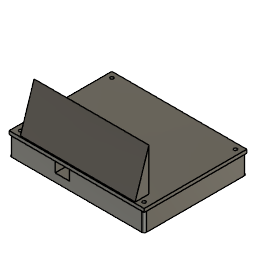
inky_case (Autodesk Fusion 360 design; units mm, degrees)
Autodesk Fusion 360 part; units mm, degrees
sketch "Sketch1" plane through (0, 0, 0) normal (0, 0, 1) x (1, 0, 0)
  line L0 (-58.8, -44.75) -> (58.8, -44.75)
  line L1 (58.8, -44.75) -> (58.8, 44.75)
  line L2 (58.8, 44.75) -> (-58.8, 44.75)
  line L3 (-58.8, 44.75) -> (-58.8, -44.75)
extrude "Extrude1" add sketch "Sketch1" along normal blind 16 makes body 1
ref_plane "WorkPlane1" through (0, 0, 2) normal (0, 0, 1) x (1, 0, 0)
sketch "Sketch2" plane through (0, 0, 2) normal (0, 0, 1) x (1, 0, 0)
  line L0 (-48.8, -34.75) -> (48.8, -34.75)
  line L1 (48.8, -34.75) -> (48.8, 34.75)
  line L2 (48.8, 34.75) -> (-48.8, 34.75)
  line L3 (-48.8, 34.75) -> (-48.8, -34.75)
extrude "Extrude2" add sketch "Sketch2" along normal blind 15 separate body makes body 2
combine "Combine1" operation cut target body 1 tool bodies 2
ref_plane "WorkPlane2" through (0, 0, -1) normal (0, 0, 1) x (1, 0, 0)
sketch "Sketch3" plane through (0, 0, -1) normal (0, 0, 1) x (1, 0, 0)
  line L0 (-43, -24.35) -> (43, -24.35)
  line L1 (43, -24.35) -> (43, 29.65)
  line L2 (43, 29.65) -> (-43, 29.65)
  line L3 (-43, 29.65) -> (-43, -24.35)
extrude "Extrude3" add sketch "Sketch3" along normal blind 4 separate body makes body 3
combine "Combine2" operation cut target body 1 tool bodies 3
ref_plane "WorkPlane3" through (0, -45.25, 0) normal (0, 1, 0) x (0, 0, 1)
sketch "Sketch4" plane through (0, -45.25, 0) normal (0, 1, 0) x (1, 0, 0)
  line L0 (-18.7, -7.2) -> (-6.3, -7.2)
  line L1 (-6.3, -7.2) -> (-6.3, -17.8)
  line L2 (-6.3, -17.8) -> (-18.7, -17.8)
  line L3 (-18.7, -17.8) -> (-18.7, -7.2)
extrude "Extrude4" add sketch "Sketch4" along normal blind 11 separate body makes body 4
combine "Combine3" operation cut target body 1 tool bodies 4
ref_plane "WorkPlane4" through (0, 0, 11) normal (0, 0, 1) x (1, 0, 0)
sketch "Sketch5" plane through (0, 0, 11) normal (0, 0, 1) x (1, 0, 0)
  circle A0 centre (-53.8, -39.75) radius 1
extrude "Extrude5" add sketch "Sketch5" along normal blind 5 separate body makes body 5
combine "Combine4" operation cut target body 1 tool bodies 5
ref_plane "WorkPlane5" through (0, 0, 11) normal (0, 0, 1) x (1, 0, 0)
sketch "Sketch6" plane through (0, 0, 11) normal (0, 0, 1) x (1, 0, 0)
  circle A0 centre (-53.8, 39.75) radius 1
extrude "Extrude6" add sketch "Sketch6" along normal blind 5 separate body makes body 6
combine "Combine5" operation cut target body 1 tool bodies 6
ref_plane "WorkPlane6" through (0, 0, 11) normal (0, 0, 1) x (1, 0, 0)
sketch "Sketch7" plane through (0, 0, 11) normal (0, 0, 1) x (1, 0, 0)
  circle A0 centre (53.8, -39.75) radius 1
extrude "Extrude7" add sketch "Sketch7" along normal blind 5 separate body makes body 7
combine "Combine6" operation cut target body 1 tool bodies 7
ref_plane "WorkPlane7" through (0, 0, 11) normal (0, 0, 1) x (1, 0, 0)
sketch "Sketch8" plane through (0, 0, 11) normal (0, 0, 1) x (1, 0, 0)
  circle A0 centre (53.8, 39.75) radius 1
extrude "Extrude8" add sketch "Sketch8" along normal blind 5 separate body makes body 8
combine "Combine7" operation cut target body 1 tool bodies 8
fillet "Fillet1" radius 2 4 edges at (-58.8, -44.75, 8) (58.8, -44.75, 8) (-58.8, 44.75, 8) (58.8, 44.75, 8) on bodies 1
ref_plane "WorkPlane8" through (0, 0, -0.5) normal (0, 0, 1) x (1, 0, 0)
sketch "Sketch9" plane through (0, 0, -0.5) normal (0, 0, 1) x (1, 0, 0)
  line L0 (-34.2331, 31.33) -> (-32.5755, 32.1283)
  line L1 (-32.5755, 32.1283) -> (-31.2436, 30.8591)
  line L2 (-31.2436, 30.8591) -> (-31.4906, 32.6823)
  line L3 (-31.4906, 32.6823) -> (-29.8719, 33.5569)
  line L4 (-29.8719, 33.5569) -> (-31.6822, 33.8853)
  line L5 (-31.6822, 33.8853) -> (-32.0138, 35.695)
  line L6 (-32.0138, 35.695) -> (-32.8856, 34.0748)
  line L7 (-32.8856, 34.0748) -> (-34.7092, 34.3187)
  line L8 (-34.7092, 34.3187) -> (-33.4377, 32.9889)
  line L9 (-33.4377, 32.9889) -> (-34.2331, 31.33)
extrude "Extrude9" add sketch "Sketch9" along normal blind 1.1 separate body makes body 9
combine "Combine8" operation cut target body 1 tool bodies 9
ref_plane "WorkPlane9" through (0, 0, -0.5) normal (0, 0, 1) x (1, 0, 0)
sketch "Sketch10" plane through (0, 0, -0.5) normal (0, 0, 1) x (1, 0, 0)
  circle A0 centre (-17.7225, 35.7912) radius 2.0607
  circle A1 centre (-16.9103, 35.6895) radius 2.0607
extrude "Extrude10" add sketch "Sketch10" along normal blind 1.1 separate body contours A0 A1 picked at (-19.4686, 36.1615) makes body 10
combine "Combine9" operation cut target body 1 tool bodies 10
ref_plane "WorkPlane10" through (0, 0, -0.5) normal (0, 0, 1) x (1, 0, 0)
sketch "Sketch11" plane through (0, 0, -0.5) normal (0, 0, 1) x (1, 0, 0)
  line L0 (-6.1051, 39.8174) -> (-6.8302, 37.9206)
  line L1 (-6.8302, 37.9206) -> (-8.853, 38.0986)
  line L2 (-8.853, 38.0986) -> (-7.2731, 36.8229)
  line L3 (-7.2731, 36.8229) -> (-8.0675, 34.954)
  line L4 (-8.0675, 34.954) -> (-6.366, 36.0624)
  line L5 (-6.366, 36.0624) -> (-4.834, 34.7294)
  line L6 (-4.834, 34.7294) -> (-5.3624, 36.6902)
  line L7 (-5.3624, 36.6902) -> (-3.6213, 37.7352)
  line L8 (-3.6213, 37.7352) -> (-5.6493, 37.8386)
  line L9 (-5.6493, 37.8386) -> (-6.1051, 39.8174)
extrude "Extrude11" add sketch "Sketch11" along normal blind 1.1 separate body makes body 11
combine "Combine10" operation cut target body 1 tool bodies 11
ref_plane "WorkPlane11" through (0, 0, -0.5) normal (0, 0, 1) x (1, 0, 0)
sketch "Sketch12" plane through (0, 0, -0.5) normal (0, 0, 1) x (1, 0, 0)
  line L0 (8.0648, 38.7951) -> (8.2392, 36.9319)
  line L1 (8.2392, 36.9319) -> (6.6062, 36.0181)
  line L2 (6.6062, 36.0181) -> (8.432, 35.6083)
  line L3 (8.432, 35.6083) -> (8.7965, 33.7728)
  line L4 (8.7965, 33.7728) -> (9.7505, 35.3826)
  line L5 (9.7505, 35.3826) -> (11.6087, 35.1621)
  line L6 (11.6087, 35.1621) -> (10.3725, 36.5669)
  line L7 (10.3725, 36.5669) -> (11.1565, 38.266)
  line L8 (11.1565, 38.266) -> (9.4385, 37.5244)
  line L9 (9.4385, 37.5244) -> (8.0648, 38.7951)
extrude "Extrude12" add sketch "Sketch12" along normal blind 1.1 separate body makes body 12
combine "Combine11" operation cut target body 1 tool bodies 12
ref_plane "WorkPlane12" through (0, 0, -0.5) normal (0, 0, 1) x (1, 0, 0)
sketch "Sketch13" plane through (0, 0, -0.5) normal (0, 0, 1) x (1, 0, 0)
  circle A0 centre (25.2651, 33.3164) radius 2.102
  circle A1 centre (24.8487, 32.1532) radius 2.102
extrude "Extrude13" add sketch "Sketch13" along normal blind 1.1 separate body contours A0 A1 picked at (26.0223, 34.8247) makes body 13
combine "Combine12" operation cut target body 1 tool bodies 13
ref_plane "WorkPlane13" through (0, 0, -0.5) normal (0, 0, 1) x (1, 0, 0)
sketch "Sketch14" plane through (0, 0, -0.5) normal (0, 0, 1) x (1, 0, 0)
  line L0 (43.3477, 37.6323) -> (44.4797, 38.9174)
  line L1 (44.4797, 38.9174) -> (46.1221, 38.4324)
  line L2 (46.1221, 38.4324) -> (45.2497, 39.9061)
  line L3 (45.2497, 39.9061) -> (46.2186, 41.3182)
  line L4 (46.2186, 41.3182) -> (44.5474, 40.9439)
  line L5 (44.5474, 40.9439) -> (43.5038, 42.3017)
  line L6 (43.5038, 42.3017) -> (43.3433, 40.5967)
  line L7 (43.3433, 40.5967) -> (41.7295, 40.0237)
  line L8 (41.7295, 40.0237) -> (43.3015, 39.3443)
  line L9 (43.3015, 39.3443) -> (43.3477, 37.6323)
extrude "Extrude14" add sketch "Sketch14" along normal blind 1.1 separate body makes body 14
combine "Combine13" operation cut target body 1 tool bodies 14
ref_plane "WorkPlane14" through (0, 0, -0.5) normal (0, 0, 1) x (1, 0, 0)
sketch "Sketch15" plane through (0, 0, -0.5) normal (0, 0, 1) x (1, 0, 0)
  line L0 (43.5729, 24.2177) -> (45.2148, 23.1167)
  line L1 (45.2148, 23.1167) -> (44.5685, 21.2483)
  line L2 (44.5685, 21.2483) -> (46.1231, 22.4697)
  line L3 (46.1231, 22.4697) -> (47.7003, 21.2777)
  line L4 (47.7003, 21.2777) -> (47.0191, 23.1336)
  line L5 (47.0191, 23.1336) -> (48.6401, 24.2652)
  line L6 (48.6401, 24.2652) -> (46.6646, 24.1909)
  line L7 (46.6646, 24.1909) -> (46.0892, 26.0823)
  line L8 (46.0892, 26.0823) -> (45.5495, 24.1804)
  line L9 (45.5495, 24.1804) -> (43.5729, 24.2177)
extrude "Extrude15" add sketch "Sketch15" along normal blind 1.1 separate body makes body 15
combine "Combine14" operation cut target body 1 tool bodies 15
ref_plane "WorkPlane15" through (0, 0, -0.5) normal (0, 0, 1) x (1, 0, 0)
sketch "Sketch16" plane through (0, 0, -0.5) normal (0, 0, 1) x (1, 0, 0)
  line L0 (53.5696, 14.8567) -> (51.5048, 15.1794)
  line L1 (51.5048, 15.1794) -> (50.9361, 17.1903)
  line L2 (50.9361, 17.1903) -> (49.9912, 15.3263)
  line L3 (49.9912, 15.3263) -> (47.903, 15.4069)
  line L4 (47.903, 15.4069) -> (49.3837, 13.9322)
  line L5 (49.3837, 13.9322) -> (48.6618, 11.9711)
  line L6 (48.6618, 11.9711) -> (50.5219, 12.9237)
  line L7 (50.5219, 12.9237) -> (52.164, 11.6311)
  line L8 (52.164, 11.6311) -> (51.8328, 13.6944)
  line L9 (51.8328, 13.6944) -> (53.5696, 14.8567)
extrude "Extrude16" add sketch "Sketch16" along normal blind 1.1 separate body makes body 16
combine "Combine15" operation cut target body 1 tool bodies 16
ref_plane "WorkPlane16" through (0, 0, -0.5) normal (0, 0, 1) x (1, 0, 0)
sketch "Sketch17" plane through (0, 0, -0.5) normal (0, 0, 1) x (1, 0, 0)
  line L0 (50.83, -3.8836) -> (49.8386, -5.605)
  line L1 (49.8386, -5.605) -> (47.9256, -5.0695)
  line L2 (47.9256, -5.0695) -> (49.2564, -6.5443)
  line L3 (49.2564, -6.5443) -> (48.1559, -8.1982)
  line L4 (48.1559, -8.1982) -> (49.9699, -7.3883)
  line L5 (49.9699, -7.3883) -> (51.2027, -8.946)
  line L6 (51.2027, -8.946) -> (50.993, -6.9706)
  line L7 (50.993, -6.9706) -> (52.8554, -6.2794)
  line L8 (52.8554, -6.2794) -> (50.9118, -5.8684)
  line L9 (50.9118, -5.8684) -> (50.83, -3.8836)
extrude "Extrude17" add sketch "Sketch17" along normal blind 1.1 separate body makes body 17
combine "Combine16" operation cut target body 1 tool bodies 17
ref_plane "WorkPlane17" through (0, 0, -0.5) normal (0, 0, 1) x (1, 0, 0)
sketch "Sketch18" plane through (0, 0, -0.5) normal (0, 0, 1) x (1, 0, 0)
  line L0 (51.6831, -25.5955) -> (53.2314, -25.8631)
  line L1 (53.2314, -25.8631) -> (53.3665, -27.4285)
  line L2 (53.3665, -27.4285) -> (54.0995, -26.0388)
  line L3 (54.0995, -26.0388) -> (55.6301, -26.3939)
  line L4 (55.6301, -26.3939) -> (54.5348, -25.2674)
  line L5 (54.5348, -25.2674) -> (55.3456, -23.9215)
  line L6 (55.3456, -23.9215) -> (53.9357, -24.615)
  line L7 (53.9357, -24.615) -> (52.9062, -23.428)
  line L8 (52.9062, -23.428) -> (53.1301, -24.9832)
  line L9 (53.1301, -24.9832) -> (51.6831, -25.5955)
extrude "Extrude18" add sketch "Sketch18" along normal blind 1.1 separate body makes body 18
combine "Combine17" operation cut target body 1 tool bodies 18
ref_plane "WorkPlane18" through (0, 0, -0.5) normal (0, 0, 1) x (1, 0, 0)
sketch "Sketch19" plane through (0, 0, -0.5) normal (0, 0, 1) x (1, 0, 0)
  line L0 (28.9464, -41.993) -> (30.4148, -41.3003)
  line L1 (30.4148, -41.3003) -> (31.5461, -42.4649)
  line L2 (31.5461, -42.4649) -> (31.3411, -40.8543)
  line L3 (31.3411, -40.8543) -> (32.7983, -40.1383)
  line L4 (32.7983, -40.1383) -> (31.2032, -39.8355)
  line L5 (31.2032, -39.8355) -> (30.9724, -38.2284)
  line L6 (30.9724, -38.2284) -> (30.1916, -39.6519)
  line L7 (30.1916, -39.6519) -> (28.5918, -39.3747)
  line L8 (28.5918, -39.3747) -> (29.7044, -40.5572)
  line L9 (29.7044, -40.5572) -> (28.9464, -41.993)
extrude "Extrude19" add sketch "Sketch19" along normal blind 1.1 separate body makes body 19
combine "Combine18" operation cut target body 1 tool bodies 19
ref_plane "WorkPlane19" through (0, 0, -0.5) normal (0, 0, 1) x (1, 0, 0)
sketch "Sketch20" plane through (0, 0, -0.5) normal (0, 0, 1) x (1, 0, 0)
  line L0 (14.6835, -35.9755) -> (16.2184, -35.1412)
  line L1 (16.2184, -35.1412) -> (17.5471, -36.2755)
  line L2 (17.5471, -36.2755) -> (17.228, -34.558)
  line L3 (17.228, -34.558) -> (18.7173, -33.6449)
  line L4 (18.7173, -33.6449) -> (16.9852, -33.4176)
  line L5 (16.9852, -33.4176) -> (16.577, -31.719)
  line L6 (16.577, -31.719) -> (15.8256, -33.2961)
  line L7 (15.8256, -33.2961) -> (14.084, -33.1594)
  line L8 (14.084, -33.1594) -> (15.3517, -34.3614)
  line L9 (15.3517, -34.3614) -> (14.6835, -35.9755)
extrude "Extrude20" add sketch "Sketch20" along normal blind 1.1 separate body makes body 20
combine "Combine19" operation cut target body 1 tool bodies 20
ref_plane "WorkPlane20" through (0, 0, -0.5) normal (0, 0, 1) x (1, 0, 0)
sketch "Sketch21" plane through (0, 0, -0.5) normal (0, 0, 1) x (1, 0, 0)
  circle A0 centre (-0.5553, -36.2656) radius 2.9824
  circle A1 centre (-0.8287, -34.7508) radius 2.9824
extrude "Extrude21" add sketch "Sketch21" along normal blind 1.1 separate body contours A0 A1 picked at (-1.201, -32.3156) makes body 21
combine "Combine20" operation cut target body 1 tool bodies 21
ref_plane "WorkPlane21" through (0, 0, -0.5) normal (0, 0, 1) x (1, 0, 0)
sketch "Sketch22" plane through (0, 0, -0.5) normal (0, 0, 1) x (1, 0, 0)
  line L0 (-9.8157, -39.8302) -> (-10.8732, -38.141)
  line L1 (-10.8732, -38.141) -> (-9.8354, -36.4397)
  line L2 (-9.8354, -36.4397) -> (-11.7686, -36.9234)
  line L3 (-11.7686, -36.9234) -> (-13.066, -35.4106)
  line L4 (-13.066, -35.4106) -> (-13.2034, -37.3987)
  line L5 (-13.2034, -37.3987) -> (-15.043, -38.1651)
  line L6 (-15.043, -38.1651) -> (-13.1946, -38.9101)
  line L7 (-13.1946, -38.9101) -> (-13.0342, -40.8966)
  line L8 (-13.0342, -40.8966) -> (-11.7545, -39.3689)
  line L9 (-11.7545, -39.3689) -> (-9.8157, -39.8302)
extrude "Extrude22" add sketch "Sketch22" along normal blind 1.1 separate body makes body 22
combine "Combine21" operation cut target body 1 tool bodies 22
ref_plane "WorkPlane22" through (0, 0, -0.5) normal (0, 0, 1) x (1, 0, 0)
sketch "Sketch23" plane through (0, 0, -0.5) normal (0, 0, 1) x (1, 0, 0)
  line L0 (-28.4961, -38.7129) -> (-29.1307, -40.2176)
  line L1 (-29.1307, -40.2176) -> (-30.7548, -40.048)
  line L2 (-30.7548, -40.048) -> (-29.5199, -41.1165)
  line L3 (-29.5199, -41.1165) -> (-30.1831, -42.6088)
  line L4 (-30.1831, -42.6088) -> (-28.7853, -41.7644)
  line L5 (-28.7853, -41.7644) -> (-27.571, -42.8563)
  line L6 (-27.571, -42.8563) -> (-27.942, -41.266)
  line L7 (-27.942, -41.266) -> (-26.5283, -40.4485)
  line L8 (-26.5283, -40.4485) -> (-28.1555, -40.31)
  line L9 (-28.1555, -40.31) -> (-28.4961, -38.7129)
extrude "Extrude23" add sketch "Sketch23" along normal blind 1.1 separate body makes body 23
combine "Combine22" operation cut target body 1 tool bodies 23
ref_plane "WorkPlane23" through (0, 0, -0.5) normal (0, 0, 1) x (1, 0, 0)
sketch "Sketch24" plane through (0, 0, -0.5) normal (0, 0, 1) x (1, 0, 0)
  line L0 (-46.7732, -24.5852) -> (-47.9706, -25.7735)
  line L1 (-47.9706, -25.7735) -> (-49.4144, -24.9011)
  line L2 (-49.4144, -24.9011) -> (-48.6542, -26.407)
  line L3 (-48.6542, -26.407) -> (-49.9301, -27.5106)
  line L4 (-49.9301, -27.5106) -> (-48.263, -27.253)
  line L5 (-48.263, -27.253) -> (-47.6077, -28.8075)
  line L6 (-47.6077, -28.8075) -> (-47.3375, -27.1423)
  line L7 (-47.3375, -27.1423) -> (-45.6566, -26.9995)
  line L8 (-45.6566, -26.9995) -> (-47.1568, -26.2279)
  line L9 (-47.1568, -26.2279) -> (-46.7732, -24.5852)
extrude "Extrude24" add sketch "Sketch24" along normal blind 1.1 separate body makes body 24
combine "Combine23" operation cut target body 1 tool bodies 24
ref_plane "WorkPlane24" through (0, 0, -0.5) normal (0, 0, 1) x (1, 0, 0)
sketch "Sketch25" plane through (0, 0, -0.5) normal (0, 0, 1) x (1, 0, 0)
  line L0 (-53.5617, -8.4744) -> (-52.2787, -9.6994)
  line L1 (-52.2787, -9.6994) -> (-52.8024, -11.3942)
  line L2 (-52.8024, -11.3942) -> (-51.2409, -10.5525)
  line L3 (-51.2409, -10.5525) -> (-49.7908, -11.5743)
  line L4 (-49.7908, -11.5743) -> (-50.1088, -9.8292)
  line L5 (-50.1088, -9.8292) -> (-48.689, -8.7658)
  line L6 (-48.689, -8.7658) -> (-50.447, -8.529)
  line L7 (-50.447, -8.529) -> (-51.0195, -6.85)
  line L8 (-51.0195, -6.85) -> (-51.788, -8.4488)
  line L9 (-51.788, -8.4488) -> (-53.5617, -8.4744)
extrude "Extrude25" add sketch "Sketch25" along normal blind 1.1 separate body makes body 25
combine "Combine24" operation cut target body 1 tool bodies 25
ref_plane "WorkPlane25" through (0, 0, -0.5) normal (0, 0, 1) x (1, 0, 0)
sketch "Sketch26" plane through (0, 0, -0.5) normal (0, 0, 1) x (1, 0, 0)
  line L0 (-49.0503, 1.275) -> (-49.0211, 3.1232)
  line L1 (-49.0211, 3.1232) -> (-47.3046, 3.809)
  line L2 (-47.3046, 3.809) -> (-49.0534, 4.4079)
  line L3 (-49.0534, 4.4079) -> (-49.1752, 6.2523)
  line L4 (-49.1752, 6.2523) -> (-50.2851, 4.7742)
  line L5 (-50.2851, 4.7742) -> (-52.0769, 5.2283)
  line L6 (-52.0769, 5.2283) -> (-51.0142, 3.7159)
  line L7 (-51.0142, 3.7159) -> (-51.9998, 2.1521)
  line L8 (-51.9998, 2.1521) -> (-50.233, 2.6956)
  line L9 (-50.233, 2.6956) -> (-49.0503, 1.275)
extrude "Extrude26" add sketch "Sketch26" along normal blind 1.1 separate body makes body 26
combine "Combine25" operation cut target body 1 tool bodies 26
ref_plane "WorkPlane26" through (0, 0, -0.5) normal (0, 0, 1) x (1, 0, 0)
sketch "Sketch27" plane through (0, 0, -0.5) normal (0, 0, 1) x (1, 0, 0)
  circle A0 centre (-46.8506, 23.0637) radius 2.848
  circle A1 centre (-45.5072, 21.712) radius 2.848
extrude "Extrude27" add sketch "Sketch27" along normal blind 1.1 separate body contours A0 A1 picked at (-48.7152, 24.2547) makes body 27
combine "Combine26" operation cut target body 1 tool bodies 27
ref_plane "WorkPlane27" through (0, 0, -0.5) normal (0, 0, 1) x (1, 0, 0)
sketch "Sketch28" plane through (0, 0, -0.5) normal (0, 0, 1) x (1, 0, 0)
  line L0 (-37.501, -43.3476) -> (-37.294, -41.6357)
  line L1 (-37.294, -41.6357) -> (-35.6131, -41.2509)
  line L2 (-35.6131, -41.2509) -> (-37.1773, -40.525)
  line L3 (-37.1773, -40.525) -> (-37.0238, -38.8075)
  line L4 (-37.0238, -38.8075) -> (-38.1975, -40.0708)
  line L5 (-38.1975, -40.0708) -> (-39.7835, -39.3941)
  line L6 (-39.7835, -39.3941) -> (-38.9448, -40.9007)
  line L7 (-38.9448, -40.9007) -> (-40.0785, -42.2)
  line L8 (-40.0785, -42.2) -> (-38.3864, -41.8679)
  line L9 (-38.3864, -41.8679) -> (-37.501, -43.3476)
extrude "Extrude28" add sketch "Sketch28" along normal blind 1.1 separate body makes body 28
combine "Combine27" operation cut target body 1 tool bodies 28
ref_plane "WorkPlane28" through (0, 0, -0.5) normal (0, 0, 1) x (1, 0, 0)
sketch "Sketch29" plane through (0, 0, -0.5) normal (0, 0, 1) x (1, 0, 0)
  circle A0 centre (-42, -35) radius 2
  circle A1 centre (-41.0474, -34.45) radius 2
extrude "Extrude29" add sketch "Sketch29" along normal blind 1.1 separate body contours A0 A1 picked at (-43.4114, -35.8148) makes body 29
combine "Combine28" operation cut target body 1 tool bodies 29
ref_plane "WorkPlane29" through (0, 0, -0.5) normal (0, 0, 1) x (1, 0, 0)
sketch "Sketch30" plane through (0, 0, -0.5) normal (0, 0, 1) x (1, 0, 0)
  line L0 (41.2584, -41.2825) -> (42.2936, -39.9035)
  line L1 (42.2936, -39.9035) -> (43.9416, -40.4107)
  line L2 (43.9416, -40.4107) -> (42.95, -39)
  line L3 (42.95, -39) -> (43.9416, -37.5893)
  line L4 (43.9416, -37.5893) -> (42.2936, -38.0965)
  line L5 (42.2936, -38.0965) -> (41.2584, -36.7175)
  line L6 (41.2584, -36.7175) -> (41.2314, -38.4416)
  line L7 (41.2314, -38.4416) -> (39.6, -39)
  line L8 (39.6, -39) -> (41.2314, -39.5584)
  line L9 (41.2314, -39.5584) -> (41.2584, -41.2825)
extrude "Extrude30" add sketch "Sketch30" along normal blind 1.1 separate body makes body 30
combine "Combine29" operation cut target body 1 tool bodies 30
ref_plane "WorkPlane30" through (0, 0, -0.5) normal (0, 0, 1) x (1, 0, 0)
sketch "Sketch31" plane through (0, 0, -0.5) normal (0, 0, 1) x (1, 0, 0)
  circle A0 centre (47, -33) radius 2
  circle A1 centre (45.9663, -33.3762) radius 2
extrude "Extrude31" add sketch "Sketch31" along normal blind 1.1 separate body contours A0 A1 picked at (48.2669, -32.8584) makes body 31
combine "Combine30" operation cut target body 1 tool bodies 31
ref_plane "WorkPlane31" through (0, 0, 16) normal (0, 0, 1) x (1, 0, 0)
sketch "Sketch32" plane through (0, 0, 16) normal (0, 0, 1) x (1, 0, 0)
  line L0 (-58.8, -44.75) -> (58.8, -44.75)
  line L1 (58.8, -44.75) -> (58.8, 44.75)
  line L2 (58.8, 44.75) -> (-58.8, 44.75)
  line L3 (-58.8, 44.75) -> (-58.8, -44.75)
extrude "Extrude32" add sketch "Sketch32" along normal blind 3 separate body makes body 32
ref_plane "WorkPlane32" through (-50, 0, 0) normal (1, 0, 0) x (0, 1, 0)
sketch "Sketch33" plane through (-50, 0, 0) normal (1, 0, 0) x (0, 0, -1)
  line L0 (-16, -44.75) -> (-16, -31.8214)
  line L1 (-16, -31.8214) -> (-56, -31.8214)
  line L2 (-56, -31.8214) -> (-16, -44.75)
extrude "Extrude33" add sketch "Sketch33" along normal blind 100 separate body makes body 33
combine "Combine31" operation add target body 32 tool bodies 33
ref_plane "WorkPlane33" through (0, 0, 15) normal (0, 0, 1) x (1, 0, 0)
sketch "Sketch34" plane through (0, 0, 15) normal (0, 0, 1) x (1, 0, 0)
  circle A0 centre (-53.8, -39.75) radius 1.4
extrude "Extrude34" add sketch "Sketch34" along normal blind 5 separate body makes body 34
combine "Combine32" operation cut target body 32 tool bodies 34
ref_plane "WorkPlane34" through (0, 0, 15) normal (0, 0, 1) x (1, 0, 0)
sketch "Sketch35" plane through (0, 0, 15) normal (0, 0, 1) x (1, 0, 0)
  circle A0 centre (-53.8, 39.75) radius 1.4
extrude "Extrude35" add sketch "Sketch35" along normal blind 5 separate body makes body 35
combine "Combine33" operation cut target body 32 tool bodies 35
ref_plane "WorkPlane35" through (0, 0, 15) normal (0, 0, 1) x (1, 0, 0)
sketch "Sketch36" plane through (0, 0, 15) normal (0, 0, 1) x (1, 0, 0)
  circle A0 centre (53.8, -39.75) radius 1.4
extrude "Extrude36" add sketch "Sketch36" along normal blind 5 separate body makes body 36
combine "Combine34" operation cut target body 32 tool bodies 36
ref_plane "WorkPlane36" through (0, 0, 15) normal (0, 0, 1) x (1, 0, 0)
sketch "Sketch37" plane through (0, 0, 15) normal (0, 0, 1) x (1, 0, 0)
  circle A0 centre (53.8, 39.75) radius 1.4
extrude "Extrude37" add sketch "Sketch37" along normal blind 5 separate body makes body 37
combine "Combine35" operation cut target body 32 tool bodies 37
ref_plane "WorkPlane37" through (0, 0, 4.5) normal (0, 0, 1) x (1, 0, 0)
sketch "Sketch38" plane through (0, 0, 4.5) normal (0, 0, 1) x (1, 0, 0)
  circle A0 centre (-44.4, -30.35) radius 3
extrude "Extrude38" add sketch "Sketch38" along normal blind 11.5 separate body makes body 38
combine "Combine36" operation add target body 32 tool bodies 38
ref_plane "WorkPlane38" through (0, 0, 4.5) normal (0, 0, 1) x (1, 0, 0)
sketch "Sketch39" plane through (0, 0, 4.5) normal (0, 0, 1) x (1, 0, 0)
  circle A0 centre (-44.4, 30.35) radius 3
extrude "Extrude39" add sketch "Sketch39" along normal blind 11.5 separate body makes body 39
combine "Combine37" operation add target body 32 tool bodies 39
ref_plane "WorkPlane39" through (0, 0, 4.5) normal (0, 0, 1) x (1, 0, 0)
sketch "Sketch40" plane through (0, 0, 4.5) normal (0, 0, 1) x (1, 0, 0)
  circle A0 centre (44.4, -30.35) radius 3
extrude "Extrude40" add sketch "Sketch40" along normal blind 11.5 separate body makes body 40
combine "Combine38" operation add target body 32 tool bodies 40
ref_plane "WorkPlane40" through (0, 0, 4.5) normal (0, 0, 1) x (1, 0, 0)
sketch "Sketch41" plane through (0, 0, 4.5) normal (0, 0, 1) x (1, 0, 0)
  circle A0 centre (44.4, 30.35) radius 3
extrude "Extrude41" add sketch "Sketch41" along normal blind 11.5 separate body makes body 41
combine "Combine39" operation add target body 32 tool bodies 41
sketch "Sketch1 (2)" plane through (0, 0, 0) normal (0, 0, 1) x (1, 0, 0) in component "Component"
  line L0 (-34.2331, 31.33) -> (-32.5755, 32.1283)
  line L1 (-32.5755, 32.1283) -> (-31.2436, 30.8591)
  line L2 (-31.2436, 30.8591) -> (-31.4906, 32.6823)
  line L3 (-31.4906, 32.6823) -> (-29.8719, 33.5569)
  line L4 (-29.8719, 33.5569) -> (-31.6822, 33.8853)
  line L5 (-31.6822, 33.8853) -> (-32.0138, 35.695)
  line L6 (-32.0138, 35.695) -> (-32.8856, 34.0748)
  line L7 (-32.8856, 34.0748) -> (-34.7092, 34.3187)
  line L8 (-34.7092, 34.3187) -> (-33.4377, 32.9889)
  line L9 (-33.4377, 32.9889) -> (-34.2331, 31.33)
extrude "Extrude1'" add sketch "Sketch1 (2)" along normal blind 0.6 separate body makes body 42 in component "Component"
sketch "Sketch2 (2)" plane through (0, 0, 0) normal (0, 0, 1) x (1, 0, 0) in component "Component"
  circle A0 centre (-17.7225, 35.7912) radius 2.0607
  circle A1 centre (-16.9103, 35.6895) radius 2.0607
extrude "Extrude2'" add sketch "Sketch2 (2)" along normal blind 0.6 separate body contours A0 A1 picked at (-19.4686, 36.1615) makes body 43 in component "Component"
sketch "Sketch3 (2)" plane through (0, 0, 0) normal (0, 0, 1) x (1, 0, 0) in component "Component"
  line L0 (-6.1051, 39.8174) -> (-6.8302, 37.9206)
  line L1 (-6.8302, 37.9206) -> (-8.853, 38.0986)
  line L2 (-8.853, 38.0986) -> (-7.2731, 36.8229)
  line L3 (-7.2731, 36.8229) -> (-8.0675, 34.954)
  line L4 (-8.0675, 34.954) -> (-6.366, 36.0624)
  line L5 (-6.366, 36.0624) -> (-4.834, 34.7294)
  line L6 (-4.834, 34.7294) -> (-5.3624, 36.6902)
  line L7 (-5.3624, 36.6902) -> (-3.6213, 37.7352)
  line L8 (-3.6213, 37.7352) -> (-5.6493, 37.8386)
  line L9 (-5.6493, 37.8386) -> (-6.1051, 39.8174)
extrude "Extrude3'" add sketch "Sketch3 (2)" along normal blind 0.6 separate body makes body 44 in component "Component"
sketch "Sketch4 (2)" plane through (0, 0, 0) normal (0, 0, 1) x (1, 0, 0) in component "Component"
  line L0 (8.0648, 38.7951) -> (8.2392, 36.9319)
  line L1 (8.2392, 36.9319) -> (6.6062, 36.0181)
  line L2 (6.6062, 36.0181) -> (8.432, 35.6083)
  line L3 (8.432, 35.6083) -> (8.7965, 33.7728)
  line L4 (8.7965, 33.7728) -> (9.7505, 35.3826)
  line L5 (9.7505, 35.3826) -> (11.6087, 35.1621)
  line L6 (11.6087, 35.1621) -> (10.3725, 36.5669)
  line L7 (10.3725, 36.5669) -> (11.1565, 38.266)
  line L8 (11.1565, 38.266) -> (9.4385, 37.5244)
  line L9 (9.4385, 37.5244) -> (8.0648, 38.7951)
extrude "Extrude4'" add sketch "Sketch4 (2)" along normal blind 0.6 separate body makes body 45 in component "Component"
sketch "Sketch5 (2)" plane through (0, 0, 0) normal (0, 0, 1) x (1, 0, 0) in component "Component"
  circle A0 centre (25.2651, 33.3164) radius 2.102
  circle A1 centre (24.8487, 32.1532) radius 2.102
extrude "Extrude5'" add sketch "Sketch5 (2)" along normal blind 0.6 separate body contours A0 A1 picked at (26.0223, 34.8247) makes body 46 in component "Component"
sketch "Sketch6 (2)" plane through (0, 0, 0) normal (0, 0, 1) x (1, 0, 0) in component "Component"
  line L0 (43.3477, 37.6323) -> (44.4797, 38.9174)
  line L1 (44.4797, 38.9174) -> (46.1221, 38.4324)
  line L2 (46.1221, 38.4324) -> (45.2497, 39.9061)
  line L3 (45.2497, 39.9061) -> (46.2186, 41.3182)
  line L4 (46.2186, 41.3182) -> (44.5474, 40.9439)
  line L5 (44.5474, 40.9439) -> (43.5038, 42.3017)
  line L6 (43.5038, 42.3017) -> (43.3433, 40.5967)
  line L7 (43.3433, 40.5967) -> (41.7295, 40.0237)
  line L8 (41.7295, 40.0237) -> (43.3015, 39.3443)
  line L9 (43.3015, 39.3443) -> (43.3477, 37.6323)
extrude "Extrude6'" add sketch "Sketch6 (2)" along normal blind 0.6 separate body makes body 47 in component "Component"
sketch "Sketch7 (2)" plane through (0, 0, 0) normal (0, 0, 1) x (1, 0, 0) in component "Component"
  line L0 (43.5729, 24.2177) -> (45.2148, 23.1167)
  line L1 (45.2148, 23.1167) -> (44.5685, 21.2483)
  line L2 (44.5685, 21.2483) -> (46.1231, 22.4697)
  line L3 (46.1231, 22.4697) -> (47.7003, 21.2777)
  line L4 (47.7003, 21.2777) -> (47.0191, 23.1336)
  line L5 (47.0191, 23.1336) -> (48.6401, 24.2652)
  line L6 (48.6401, 24.2652) -> (46.6646, 24.1909)
  line L7 (46.6646, 24.1909) -> (46.0892, 26.0823)
  line L8 (46.0892, 26.0823) -> (45.5495, 24.1804)
  line L9 (45.5495, 24.1804) -> (43.5729, 24.2177)
extrude "Extrude7'" add sketch "Sketch7 (2)" along normal blind 0.6 separate body makes body 48 in component "Component"
sketch "Sketch8 (2)" plane through (0, 0, 0) normal (0, 0, 1) x (1, 0, 0) in component "Component"
  line L0 (53.5696, 14.8567) -> (51.5048, 15.1794)
  line L1 (51.5048, 15.1794) -> (50.9361, 17.1903)
  line L2 (50.9361, 17.1903) -> (49.9912, 15.3263)
  line L3 (49.9912, 15.3263) -> (47.903, 15.4069)
  line L4 (47.903, 15.4069) -> (49.3837, 13.9322)
  line L5 (49.3837, 13.9322) -> (48.6618, 11.9711)
  line L6 (48.6618, 11.9711) -> (50.5219, 12.9237)
  line L7 (50.5219, 12.9237) -> (52.164, 11.6311)
  line L8 (52.164, 11.6311) -> (51.8328, 13.6944)
  line L9 (51.8328, 13.6944) -> (53.5696, 14.8567)
extrude "Extrude8'" add sketch "Sketch8 (2)" along normal blind 0.6 separate body makes body 49 in component "Component"
sketch "Sketch9 (2)" plane through (0, 0, 0) normal (0, 0, 1) x (1, 0, 0) in component "Component"
  line L0 (50.83, -3.8836) -> (49.8386, -5.605)
  line L1 (49.8386, -5.605) -> (47.9256, -5.0695)
  line L2 (47.9256, -5.0695) -> (49.2564, -6.5443)
  line L3 (49.2564, -6.5443) -> (48.1559, -8.1982)
  line L4 (48.1559, -8.1982) -> (49.9699, -7.3883)
  line L5 (49.9699, -7.3883) -> (51.2027, -8.946)
  line L6 (51.2027, -8.946) -> (50.993, -6.9706)
  line L7 (50.993, -6.9706) -> (52.8554, -6.2794)
  line L8 (52.8554, -6.2794) -> (50.9118, -5.8684)
  line L9 (50.9118, -5.8684) -> (50.83, -3.8836)
extrude "Extrude9'" add sketch "Sketch9 (2)" along normal blind 0.6 separate body makes body 50 in component "Component"
sketch "Sketch10 (2)" plane through (0, 0, 0) normal (0, 0, 1) x (1, 0, 0) in component "Component"
  line L0 (51.6831, -25.5955) -> (53.2314, -25.8631)
  line L1 (53.2314, -25.8631) -> (53.3665, -27.4285)
  line L2 (53.3665, -27.4285) -> (54.0995, -26.0388)
  line L3 (54.0995, -26.0388) -> (55.6301, -26.3939)
  line L4 (55.6301, -26.3939) -> (54.5348, -25.2674)
  line L5 (54.5348, -25.2674) -> (55.3456, -23.9215)
  line L6 (55.3456, -23.9215) -> (53.9357, -24.615)
  line L7 (53.9357, -24.615) -> (52.9062, -23.428)
  line L8 (52.9062, -23.428) -> (53.1301, -24.9832)
  line L9 (53.1301, -24.9832) -> (51.6831, -25.5955)
extrude "Extrude10'" add sketch "Sketch10 (2)" along normal blind 0.6 separate body makes body 51 in component "Component"
sketch "Sketch11 (2)" plane through (0, 0, 0) normal (0, 0, 1) x (1, 0, 0) in component "Component"
  line L0 (28.9464, -41.993) -> (30.4148, -41.3003)
  line L1 (30.4148, -41.3003) -> (31.5461, -42.4649)
  line L2 (31.5461, -42.4649) -> (31.3411, -40.8543)
  line L3 (31.3411, -40.8543) -> (32.7983, -40.1383)
  line L4 (32.7983, -40.1383) -> (31.2032, -39.8355)
  line L5 (31.2032, -39.8355) -> (30.9724, -38.2284)
  line L6 (30.9724, -38.2284) -> (30.1916, -39.6519)
  line L7 (30.1916, -39.6519) -> (28.5918, -39.3747)
  line L8 (28.5918, -39.3747) -> (29.7044, -40.5572)
  line L9 (29.7044, -40.5572) -> (28.9464, -41.993)
extrude "Extrude11'" add sketch "Sketch11 (2)" along normal blind 0.6 separate body makes body 52 in component "Component"
sketch "Sketch12 (2)" plane through (0, 0, 0) normal (0, 0, 1) x (1, 0, 0) in component "Component"
  line L0 (14.6835, -35.9755) -> (16.2184, -35.1412)
  line L1 (16.2184, -35.1412) -> (17.5471, -36.2755)
  line L2 (17.5471, -36.2755) -> (17.228, -34.558)
  line L3 (17.228, -34.558) -> (18.7173, -33.6449)
  line L4 (18.7173, -33.6449) -> (16.9852, -33.4176)
  line L5 (16.9852, -33.4176) -> (16.577, -31.719)
  line L6 (16.577, -31.719) -> (15.8256, -33.2961)
  line L7 (15.8256, -33.2961) -> (14.084, -33.1594)
  line L8 (14.084, -33.1594) -> (15.3517, -34.3614)
  line L9 (15.3517, -34.3614) -> (14.6835, -35.9755)
extrude "Extrude12'" add sketch "Sketch12 (2)" along normal blind 0.6 separate body makes body 53 in component "Component"
sketch "Sketch13 (2)" plane through (0, 0, 0) normal (0, 0, 1) x (1, 0, 0) in component "Component"
  circle A0 centre (-0.5553, -36.2656) radius 2.9824
  circle A1 centre (-0.8287, -34.7508) radius 2.9824
extrude "Extrude13'" add sketch "Sketch13 (2)" along normal blind 0.6 separate body contours A0 A1 picked at (-1.201, -32.3156) makes body 54 in component "Component"
sketch "Sketch14 (2)" plane through (0, 0, 0) normal (0, 0, 1) x (1, 0, 0) in component "Component"
  line L0 (-9.8157, -39.8302) -> (-10.8732, -38.141)
  line L1 (-10.8732, -38.141) -> (-9.8354, -36.4397)
  line L2 (-9.8354, -36.4397) -> (-11.7686, -36.9234)
  line L3 (-11.7686, -36.9234) -> (-13.066, -35.4106)
  line L4 (-13.066, -35.4106) -> (-13.2034, -37.3987)
  line L5 (-13.2034, -37.3987) -> (-15.043, -38.1651)
  line L6 (-15.043, -38.1651) -> (-13.1946, -38.9101)
  line L7 (-13.1946, -38.9101) -> (-13.0342, -40.8966)
  line L8 (-13.0342, -40.8966) -> (-11.7545, -39.3689)
  line L9 (-11.7545, -39.3689) -> (-9.8157, -39.8302)
extrude "Extrude14'" add sketch "Sketch14 (2)" along normal blind 0.6 separate body makes body 55 in component "Component"
sketch "Sketch15 (2)" plane through (0, 0, 0) normal (0, 0, 1) x (1, 0, 0) in component "Component"
  line L0 (-28.4961, -38.7129) -> (-29.1307, -40.2176)
  line L1 (-29.1307, -40.2176) -> (-30.7548, -40.048)
  line L2 (-30.7548, -40.048) -> (-29.5199, -41.1165)
  line L3 (-29.5199, -41.1165) -> (-30.1831, -42.6088)
  line L4 (-30.1831, -42.6088) -> (-28.7853, -41.7644)
  line L5 (-28.7853, -41.7644) -> (-27.571, -42.8563)
  line L6 (-27.571, -42.8563) -> (-27.942, -41.266)
  line L7 (-27.942, -41.266) -> (-26.5283, -40.4485)
  line L8 (-26.5283, -40.4485) -> (-28.1555, -40.31)
  line L9 (-28.1555, -40.31) -> (-28.4961, -38.7129)
extrude "Extrude15'" add sketch "Sketch15 (2)" along normal blind 0.6 separate body makes body 56 in component "Component"
sketch "Sketch16 (2)" plane through (0, 0, 0) normal (0, 0, 1) x (1, 0, 0) in component "Component"
  line L0 (-46.7732, -24.5852) -> (-47.9706, -25.7735)
  line L1 (-47.9706, -25.7735) -> (-49.4144, -24.9011)
  line L2 (-49.4144, -24.9011) -> (-48.6542, -26.407)
  line L3 (-48.6542, -26.407) -> (-49.9301, -27.5106)
  line L4 (-49.9301, -27.5106) -> (-48.263, -27.253)
  line L5 (-48.263, -27.253) -> (-47.6077, -28.8075)
  line L6 (-47.6077, -28.8075) -> (-47.3375, -27.1423)
  line L7 (-47.3375, -27.1423) -> (-45.6566, -26.9995)
  line L8 (-45.6566, -26.9995) -> (-47.1568, -26.2279)
  line L9 (-47.1568, -26.2279) -> (-46.7732, -24.5852)
extrude "Extrude16'" add sketch "Sketch16 (2)" along normal blind 0.6 separate body makes body 57 in component "Component"
sketch "Sketch17 (2)" plane through (0, 0, 0) normal (0, 0, 1) x (1, 0, 0) in component "Component"
  line L0 (-53.5617, -8.4744) -> (-52.2787, -9.6994)
  line L1 (-52.2787, -9.6994) -> (-52.8024, -11.3942)
  line L2 (-52.8024, -11.3942) -> (-51.2409, -10.5525)
  line L3 (-51.2409, -10.5525) -> (-49.7908, -11.5743)
  line L4 (-49.7908, -11.5743) -> (-50.1088, -9.8292)
  line L5 (-50.1088, -9.8292) -> (-48.689, -8.7658)
  line L6 (-48.689, -8.7658) -> (-50.447, -8.529)
  line L7 (-50.447, -8.529) -> (-51.0195, -6.85)
  line L8 (-51.0195, -6.85) -> (-51.788, -8.4488)
  line L9 (-51.788, -8.4488) -> (-53.5617, -8.4744)
extrude "Extrude17'" add sketch "Sketch17 (2)" along normal blind 0.6 separate body makes body 58 in component "Component"
sketch "Sketch18 (2)" plane through (0, 0, 0) normal (0, 0, 1) x (1, 0, 0) in component "Component"
  line L0 (-49.0503, 1.275) -> (-49.0211, 3.1232)
  line L1 (-49.0211, 3.1232) -> (-47.3046, 3.809)
  line L2 (-47.3046, 3.809) -> (-49.0534, 4.4079)
  line L3 (-49.0534, 4.4079) -> (-49.1752, 6.2523)
  line L4 (-49.1752, 6.2523) -> (-50.2851, 4.7742)
  line L5 (-50.2851, 4.7742) -> (-52.0769, 5.2283)
  line L6 (-52.0769, 5.2283) -> (-51.0142, 3.7159)
  line L7 (-51.0142, 3.7159) -> (-51.9998, 2.1521)
  line L8 (-51.9998, 2.1521) -> (-50.233, 2.6956)
  line L9 (-50.233, 2.6956) -> (-49.0503, 1.275)
extrude "Extrude18'" add sketch "Sketch18 (2)" along normal blind 0.6 separate body makes body 59 in component "Component"
sketch "Sketch19 (2)" plane through (0, 0, 0) normal (0, 0, 1) x (1, 0, 0) in component "Component"
  circle A0 centre (-46.8506, 23.0637) radius 2.848
  circle A1 centre (-45.5072, 21.712) radius 2.848
extrude "Extrude19'" add sketch "Sketch19 (2)" along normal blind 0.6 separate body contours A0 A1 picked at (-48.7152, 24.2547) makes body 60 in component "Component"
sketch "Sketch20 (2)" plane through (0, 0, 0) normal (0, 0, 1) x (1, 0, 0) in component "Component"
  line L0 (-37.501, -43.3476) -> (-37.294, -41.6357)
  line L1 (-37.294, -41.6357) -> (-35.6131, -41.2509)
  line L2 (-35.6131, -41.2509) -> (-37.1773, -40.525)
  line L3 (-37.1773, -40.525) -> (-37.0238, -38.8075)
  line L4 (-37.0238, -38.8075) -> (-38.1975, -40.0708)
  line L5 (-38.1975, -40.0708) -> (-39.7835, -39.3941)
  line L6 (-39.7835, -39.3941) -> (-38.9448, -40.9007)
  line L7 (-38.9448, -40.9007) -> (-40.0785, -42.2)
  line L8 (-40.0785, -42.2) -> (-38.3864, -41.8679)
  line L9 (-38.3864, -41.8679) -> (-37.501, -43.3476)
extrude "Extrude20'" add sketch "Sketch20 (2)" along normal blind 0.6 separate body makes body 61 in component "Component"
sketch "Sketch21 (2)" plane through (0, 0, 0) normal (0, 0, 1) x (1, 0, 0) in component "Component"
  circle A0 centre (-42, -35) radius 2
  circle A1 centre (-41.0474, -34.45) radius 2
extrude "Extrude21'" add sketch "Sketch21 (2)" along normal blind 0.6 separate body contours A0 A1 picked at (-43.4114, -35.8148) makes body 62 in component "Component"
sketch "Sketch22 (2)" plane through (0, 0, 0) normal (0, 0, 1) x (1, 0, 0) in component "Component"
  line L0 (41.2584, -41.2825) -> (42.2936, -39.9035)
  line L1 (42.2936, -39.9035) -> (43.9416, -40.4107)
  line L2 (43.9416, -40.4107) -> (42.95, -39)
  line L3 (42.95, -39) -> (43.9416, -37.5893)
  line L4 (43.9416, -37.5893) -> (42.2936, -38.0965)
  line L5 (42.2936, -38.0965) -> (41.2584, -36.7175)
  line L6 (41.2584, -36.7175) -> (41.2314, -38.4416)
  line L7 (41.2314, -38.4416) -> (39.6, -39)
  line L8 (39.6, -39) -> (41.2314, -39.5584)
  line L9 (41.2314, -39.5584) -> (41.2584, -41.2825)
extrude "Extrude22'" add sketch "Sketch22 (2)" along normal blind 0.6 separate body makes body 63 in component "Component"
sketch "Sketch23 (2)" plane through (0, 0, 0) normal (0, 0, 1) x (1, 0, 0) in component "Component"
  circle A0 centre (47, -33) radius 2
  circle A1 centre (45.9663, -33.3762) radius 2
extrude "Extrude23'" add sketch "Sketch23 (2)" along normal blind 0.6 separate body contours A0 A1 picked at (48.2669, -32.8584) makes body 64 in component "Component"
component "Component" placed x (1, 0, 0) y (0, 1, 0) z (0, 0, 1) at (0, 0, 0)
